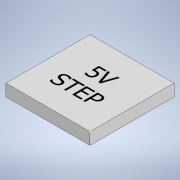
# Autodesk Inventor part: 5V_step
Saved by Autodesk Inventor 2020 (Build 240168000, 168)
## iProperties
Created: 2019-10-29
Part Number: 5V_step
Material: Generic
Document SubType Name: Modeling
Designer: Connor
Density: 1 g/cm^3
Appearance: Default
Author: Connor
Autodesk Inventor part; units mm, degrees
ref_plane "YZ Plane" through (0, 0, 0) normal (1, 0, 0) x (0, 1, 0)
ref_plane "XZ Plane" through (0, 0, 0) normal (0, 1, 0) x (-1, 0, 0)
ref_plane "XY Plane" through (0, 0, 0) normal (0, 0, 1) x (1, 0, 0)
sketch "Sketch1" plane through (0, 0, 0) normal (0, 1, 0) x (-1, 0, 0)
  line L0 (0, 0) -> (17.78, 0)
  line L1 (17.78, 0) -> (17.78, -17.78)
  line L2 (17.78, -17.78) -> (0, -17.78)
  line L3 (0, -17.78) -> (0, 0)
  dimension "d0" = 17.78
  dimension "d1" = 17.78
  constraints: 8 end point, 2 parallel, 1 horizontal, 1 perpendicular
  measures "d0" distance of L1.end L2.end
  measures "d1" distance of L0.end L1.end
extrude "Extrusion1" add sketch "Sketch1" along normal blind 2.54
sketch "Sketch2" plane through (0, 2.54, 0) normal (0, 1, 0) x (1, 0, 0)
  line L0 (-14.7493, 12.9832) -> (-3.389, 12.9832) construction
  line L1 (-3.389, 12.9832) -> (-3.389, 3.2458) construction
  line L2 (-3.389, 3.2458) -> (-14.7493, 3.2458) construction
  line L3 (-14.7493, 3.2458) -> (-14.7493, 12.9832) construction
  point P0 (0, 0)
  constraints: 2 other
body "Solid1"
